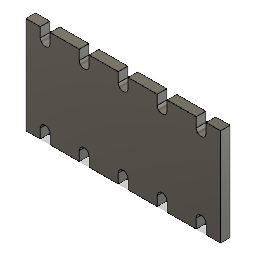
Table_17p1_Problem_19 (Autodesk Fusion 360 design; units mm, degrees)
Autodesk Fusion 360 part; units mm, degrees
sketch "Sketch1" plane through (0, 0, 0) normal (0, 0, 1) x (1, 0, 0)
  line L0 (-10, 25) -> (-2.5, 25)
  line L1 (-2.5, 25) -> (-2.5, 20)
  arc A0 (-2.5, 20) -> (0, 17.5) centre (0, 20) ccw
  arc A1 (0, 17.5) -> (2.5, 20) centre (0, 20) ccw
  line L2 (2.5, 20) -> (2.5, 25)
  line L3 (2.5, 25) -> (10, 25)
  line L4 (0, 0) -> (0, 20) construction
  line L5 (0, 0) -> (10, 0) construction
  line L6 (-10, -25) -> (-2.5, -25)
  line L7 (-2.5, -25) -> (-2.5, -20)
  arc A2 (0, -17.5) -> (-2.5, -20) centre (0, -20) ccw
  arc A3 (2.5, -20) -> (0, -17.5) centre (0, -20) ccw
  line L8 (2.5, -20) -> (2.5, -25)
  line L9 (2.5, -25) -> (10, -25)
  line L10 (10, -25) -> (10, 25)
  line L11 (-10, -25) -> (-10, 25)
  line L12 (-10, 17.5) -> (10, 17.5) construction
  line L13 (-37.5, 25) -> (-30, 25)
  line L14 (-37.5, 20) -> (-37.5, 25)
  arc A4 (-40, 17.5) -> (-37.5, 20) centre (-40, 20) ccw
  arc A5 (-42.5, 20) -> (-40, 17.5) centre (-40, 20) ccw
  line L15 (-42.5, 25) -> (-42.5, 20)
  line L16 (-50, 25) -> (-42.5, 25)
  line L17 (-50, -25) -> (-50, 25)
  line L18 (-50, -25) -> (-42.5, -25)
  line L19 (-42.5, -25) -> (-42.5, -20)
  arc A6 (-40, -17.5) -> (-42.5, -20) centre (-40, -20) ccw
  arc A7 (-37.5, -20) -> (-40, -17.5) centre (-40, -20) ccw
  line L20 (-37.5, -20) -> (-37.5, -25)
  line L21 (-37.5, -25) -> (-30, -25)
  line L22 (-30, -25) -> (-30, 25)
  line L23 (-17.5, 25) -> (-10, 25)
  line L24 (-17.5, 20) -> (-17.5, 25)
  arc A8 (-20, 17.5) -> (-17.5, 20) centre (-20, 20) ccw
  arc A9 (-22.5, 20) -> (-20, 17.5) centre (-20, 20) ccw
  line L25 (-22.5, 25) -> (-22.5, 20)
  line L26 (-30, 25) -> (-22.5, 25)
  line L27 (-30, -25) -> (-30, 25)
  line L28 (-30, -25) -> (-22.5, -25)
  line L29 (-22.5, -25) -> (-22.5, -20)
  arc A10 (-20, -17.5) -> (-22.5, -20) centre (-20, -20) ccw
  arc A11 (-17.5, -20) -> (-20, -17.5) centre (-20, -20) ccw
  line L30 (-17.5, -20) -> (-17.5, -25)
  line L31 (-17.5, -25) -> (-10, -25)
  line L32 (-10, -25) -> (-10, 25)
  line L33 (22.5, 25) -> (30, 25)
  line L34 (22.5, 20) -> (22.5, 25)
  arc A12 (20, 17.5) -> (22.5, 20) centre (20, 20) ccw
  arc A13 (17.5, 20) -> (20, 17.5) centre (20, 20) ccw
  line L35 (17.5, 25) -> (17.5, 20)
  line L36 (10, 25) -> (17.5, 25)
  line L37 (10, -25) -> (10, 25)
  line L38 (10, -25) -> (17.5, -25)
  line L39 (17.5, -25) -> (17.5, -20)
  arc A14 (20, -17.5) -> (17.5, -20) centre (20, -20) ccw
  arc A15 (22.5, -20) -> (20, -17.5) centre (20, -20) ccw
  line L40 (22.5, -20) -> (22.5, -25)
  line L41 (22.5, -25) -> (30, -25)
  line L42 (30, -25) -> (30, 25)
  line L43 (42.5, 25) -> (50, 25)
  line L44 (42.5, 20) -> (42.5, 25)
  arc A16 (40, 17.5) -> (42.5, 20) centre (40, 20) ccw
  arc A17 (37.5, 20) -> (40, 17.5) centre (40, 20) ccw
  line L45 (37.5, 25) -> (37.5, 20)
  line L46 (30, 25) -> (37.5, 25)
  line L47 (30, -25) -> (30, 25)
  line L48 (30, -25) -> (37.5, -25)
  line L49 (37.5, -25) -> (37.5, -20)
  arc A18 (40, -17.5) -> (37.5, -20) centre (40, -20) ccw
  arc A19 (42.5, -20) -> (40, -17.5) centre (40, -20) ccw
  line L50 (42.5, -20) -> (42.5, -25)
  line L51 (42.5, -25) -> (50, -25)
  line L52 (50, -25) -> (50, 25)
  dimension "Notch_Radius" = 2.5
  dimension "Notch_Height" = 7.5
  dimension "Total_Height" = 50
  dimension "Repeat_Length" = 20
  dimension "Repeat_Spacing" = 20
  dimension "d8" = 0
  constraint coincident L4.start L5.start
  constraint horizontal L0
  constraint perpendicular L0 L1
  constraint tangent L1 A0
  constraint tangent A0 A1
  constraint parallel L1 L2
  constraint perpendicular L1 L3
  constraint equal L0 L3
  constraint equal L1 L2
  constraint equal A0 A1
  constraint tangent A1 L2
  constraint coincident A0.centre A1.centre
  constraint vertical L4
  constraint perpendicular L4 L5
  constraint symmetric L0.start L5 L6.start
  constraint symmetric L0.end L5 L6.end
  constraint symmetric L1.end L5 L7.end
  constraint symmetric A0.end L5 A2.start
  constraint symmetric A0 L5 A2
  constraint symmetric A1.end L5 A3.start
  constraint symmetric A1 L5 A3
  constraint symmetric L2.end L5 L8.end
  constraint symmetric L3.end L5 L9.end
  constraint coincident L5.end L10
  constraint coincident A0.end L4
  constraint coincident L11 L12.start
  constraint coincident L10 L12.end
  constraint perpendicular L10 L12
  constraint tangent A1 L12
  measures "Notch_Radius" radius of A1
  measures "Notch_Height" distance of L3 L12
  measures "Total_Height" distance of L3.end L9.end
  measures "Repeat_Length" distance of L10 L11
extrude "Extrude1" add sketch "Sketch1" along normal mid plane 5
equation "Number_Repeat = 5"
equation "Thickness = 0.5 cm"
